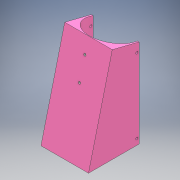
# Autodesk Inventor part: rampe-goulotte
Saved by Autodesk Inventor 2017 (Build 210142000, 142)
## iProperties
Created: 2018-04-06
Part Number: rampe-goulotte
Material: Generic
Document SubType Name: Modeling
Designer: franc
Density: 1 g/cm^3
Appearance: Default
Author: franc
Autodesk Inventor part; units mm, degrees
ref_plane "YZ Plane" through (0, 0, 0) normal (1, 0, 0) x (0, 1, 0)
ref_plane "XZ Plane" through (0, 0, 0) normal (0, 1, 0) x (-1, 0, 0)
ref_plane "XY Plane" through (0, 0, 0) normal (0, 0, 1) x (1, 0, 0)
sketch "Sketch1" plane through (0, 0, 0) normal (0, 1, 0) x (-1, 0, 0)
  line L0 (23.8582, 45.9592) -> (-40.1418, 45.9592)
  line L1 (-40.1418, 45.9592) -> (-40.1418, -94.0408)
  line L2 (-40.1418, -94.0408) -> (23.8582, -94.0408)
  line L3 (23.8582, -94.0408) -> (23.8582, 45.9592)
  point P0 (0, 0)
  dimension "d0" = 140
  dimension "d1" = 64
  constraints: 8 end point, 2 parallel, 1 horizontal, 1 perpendicular
  measures "d0" distance of L2.end L0.start
  measures "d1" distance of L0.start L0.end
extrude "Extrusion1" add sketch "Sketch1" along normal blind 36
sketch "Sketch2" plane through (40.1418, 0, 45.9592) normal (1, 0, 0) x (0, 0, -1)
  line L0 (0, 0) -> (140, 0) projected
  line L1 (0, 36) -> (140, 36) projected
  line L2 (0, 0) -> (0, 36)
  line L3 (140, 0) -> (0, 35)
  line L4 (0, 0) -> (0, 36) projected
  point P0 (45.9592, 0)
  dimension "d35" = 1
  constraints: 4 end point, 1 point on line, 1 vertical
  measures "d35" distance from line of L1 L3.end
extrude "Extrusion2" cut sketch "Sketch2" against normal through all
sketch "Sketch5" plane through (40.1418, 36, -94.0408) normal (0, 0, -1) x (-1, 0, 0)
  line L0 (64, 0) -> (0, 0)
  line L1 (0, 0) -> (0, 35)
  line L2 (0, 35) -> (64, 35)
  line L3 (64, 35) -> (64, 0)
  line L4 (64, -36) -> (64, 0) projected
  line L5 (0, -36) -> (0, 0) projected
  line L6 (0, 0) -> (64, 0) projected
  point P0 (40.1418, -36)
  dimension "d18" = 0
  dimension "d19" = 0
  dimension "d20" = 35
  dimension "d23" = 0
  constraints: 8 end point, 2 parallel, 1 horizontal, 1 perpendicular
  measures "d18" distance between parallel lines of L4 L3
  measures "d19" distance between parallel lines of L5 L1
  measures "d20" distance of L0.end L1.end
  measures "d23" distance between parallel lines of L6 L0
extrude "Extrusion3" add sketch "Sketch5" against normal blind 140
sketch "Sketch8" plane through (40.1418, 0, -94.0408) normal (0, 0, -1) x (-1, 0, 0)
  circle A0 centre (32, 66) radius 30
  line L0 (0, 0) -> (64, 0) projected
  line L1 (0, 0) -> (0, 71) projected
  point P0 (40.1418, 0)
  dimension "d43" = 66
  dimension "d44" = 32
  dimension "d45" = 60
  constraints: 1 centre point
  measures "d43" distance from line of L0 A0.centre
  measures "d44" distance from line of L1 A0.centre
  measures "d45" diameter of A0
extrude "Extrusion6" cut sketch "Sketch8" against normal through all
sketch "Sketch9" plane through (-23.8582, 0, -94.0408) normal (-1, 0, 0) x (0, 0, 1)
  circle A0 centre (20, 68) radius 1.5
  circle A1 centre (120, 68) radius 1.5
  line L0 (0, 0) -> (0, 71) projected
  line L1 (0, 71) -> (140, 71) projected
  point P0 (94.0408, 0)
  dimension "d48" = 20
  dimension "d49" = 3
  dimension "d50" = 3
  dimension "d51" = 3
  dimension "d52" = 3
  dimension "d53" = 120
  constraints: 2 centre point
  measures "d48" distance from line of A0.centre L0
  measures "d49" distance from line of L1 A0.centre
  measures "d50" diameter of A0
  measures "d51" distance from line of L1 A1.centre
  measures "d52" diameter of A1
  measures "d53" distance from line of L0 A1.centre
extrude "Extrusion7" cut sketch "Sketch9" against normal through all
sketch "Sketch10" plane through (-23.8582, 0, -94.0408) normal (-1, 0, 0) x (0, 0, 1)
  line L0 (140, 35) -> (140, 71) projected
  line L1 (140, 35) -> (131, 71)
  line L2 (0, 0) -> (140, 35) projected
  line L3 (140, 71) -> (131, 71)
  line L4 (0, 71) -> (140, 71) projected
  line L5 (140, 71) -> (0, 71) projected
  line L6 (12, 71) -> (12, 3)
  line L7 (0, 0) -> (0, 71) projected
  point P0 (94.0408, 0)
  dimension "d56" = 90
  dimension "d67" = 12
  constraints: 6 end point, 3 point on line, 1 vertical
  measures "d56" angle of L2 L1
  measures "d67" distance between parallel lines of L7 L6
extrude "Extrusion8" cut sketch "Sketch10" against normal through all contours L1 L3 L0 | L2 L7 L4 L6
sketch "Sketch11" plane through (-23.8582, 0, -94.0408) normal (0, -0.9701425, 0.2425356) x (1, 0, 0)
  circle A0 centre (32, 124.3087) radius 1.5
  line L0 (0, 0) -> (0, 144.3087) projected
  line L1 (0, 144.3087) -> (64, 144.3087) projected
  circle A1 centre (32, 94.3087) radius 1.5
  point P0 (23.8582, 91.2329)
  dimension "d59" = 3
  dimension "d60" = 32
  dimension "d61" = 20
  dimension "d62" = 32
  dimension "d63" = 50
  dimension "d64" = 3
  constraints: 2 centre point
  measures "d59" diameter of A0
  measures "d60" distance from line of L0 A0.centre
  measures "d61" distance from line of L1 A0.centre
  measures "d62" distance from line of L0 A1.centre
  measures "d63" distance from line of L1 A1.centre
  measures "d64" diameter of A1
extrude "Extrusion9" cut sketch "Sketch11" against normal through all
body "Solid1"
